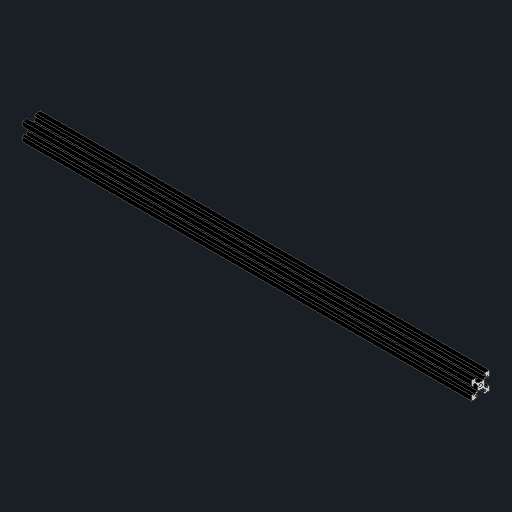
# Autodesk Inventor part: V Extrustion 20x500mm
Saved by Autodesk Inventor 2025.1 (Build 291241000, 241)
## iProperties
Created: 2024-10-17
Part Number: V Extrustion 20x500mm
Material: Generic
Document SubType Name: Modeling
Designer: jerem
Density: 1 g/cm^3
Appearance: Default
Author: jerem
Autodesk Inventor part; units mm, degrees
ref_plane "YZ Plane" through (0, 0, 0) normal (1, 0, 0) x (0, 1, 0)
ref_plane "XZ Plane" through (0, 0, 0) normal (0, 1, 0) x (-1, 0, 0)
ref_plane "XY Plane" through (0, 0, 0) normal (0, 0, 1) x (1, 0, 0)
sketch "Sketch1" plane through (0, 0, 0) normal (1, 0, 0) x (0, 1, 0)
  line L0 (-9.95, -9.95) -> (9.95, -9.95) construction
  line L1 (9.95, 9.95) -> (-9.95, 9.95) construction
  line L2 (-9.95, 9.95) -> (-9.95, -9.95) construction
  line L3 (-9.95, -9.95) -> (9.95, 9.95) construction
  line L4 (9.95, -9.95) -> (-9.95, 9.95) construction
  line L5 (9.95, 4.925) -> (8.15, 3.125)
  line L6 (8.15, 3.125) -> (8.15, 5.4393)
  line L7 (8.15, 5.4393) -> (6.5, 5.4393)
  line L8 (6.5, 5.4393) -> (3.9107, 2.85)
  line L9 (3.9107, 2.85) -> (3.9107, 0)
  line L10 (9.95, -4.925) -> (8.15, -3.125)
  line L11 (8.15, -3.125) -> (8.15, -5.4393)
  line L12 (3.9107, -2.85) -> (3.9107, 0)
  line L13 (0, 0) -> (6.8658, 0) construction
  line L14 (8.15, -5.4393) -> (6.5, -5.4393)
  line L15 (6.5, -5.4393) -> (3.9107, -2.85)
  circle A0 centre (0, 0) radius 2
  line L16 (9.95, -9.95) -> (9.95, -4.925)
  line L17 (9.95, 4.925) -> (9.95, 9.95)
  line L18 (-4.925, 9.95) -> (-9.95, 9.95)
  line L19 (-4.925, 9.95) -> (-3.125, 8.15)
  line L20 (-5.4393, 6.5) -> (-2.85, 3.9107)
  line L21 (-5.4393, 8.15) -> (-5.4393, 6.5)
  line L22 (-3.125, 8.15) -> (-5.4393, 8.15)
  line L23 (-2.85, 3.9107) -> (0, 3.9107)
  line L24 (2.85, 3.9107) -> (0, 3.9107)
  line L25 (5.4393, 6.5) -> (2.85, 3.9107)
  line L26 (5.4393, 8.15) -> (5.4393, 6.5)
  line L27 (3.125, 8.15) -> (5.4393, 8.15)
  line L28 (4.925, 9.95) -> (3.125, 8.15)
  line L29 (9.95, 9.95) -> (4.925, 9.95)
  line L30 (-9.95, -4.925) -> (-9.95, -9.95)
  line L31 (-9.95, -4.925) -> (-8.15, -3.125)
  line L32 (-6.5, -5.4393) -> (-3.9107, -2.85)
  line L33 (-8.15, -5.4393) -> (-6.5, -5.4393)
  line L34 (-8.15, -3.125) -> (-8.15, -5.4393)
  line L35 (-3.9107, -2.85) -> (-3.9107, 0)
  line L36 (-3.9107, 2.85) -> (-3.9107, 0)
  line L37 (-6.5, 5.4393) -> (-3.9107, 2.85)
  line L38 (-8.15, 5.4393) -> (-6.5, 5.4393)
  line L39 (-8.15, 3.125) -> (-8.15, 5.4393)
  line L40 (-9.95, 4.925) -> (-8.15, 3.125)
  line L41 (-9.95, 9.95) -> (-9.95, 4.925)
  line L42 (4.925, -9.95) -> (9.95, -9.95)
  line L43 (4.925, -9.95) -> (3.125, -8.15)
  line L44 (5.4393, -6.5) -> (2.85, -3.9107)
  line L45 (5.4393, -8.15) -> (5.4393, -6.5)
  line L46 (3.125, -8.15) -> (5.4393, -8.15)
  line L47 (2.85, -3.9107) -> (0, -3.9107)
  line L48 (-2.85, -3.9107) -> (0, -3.9107)
  line L49 (-5.4393, -6.5) -> (-2.85, -3.9107)
  line L50 (-5.4393, -8.15) -> (-5.4393, -6.5)
  line L51 (-3.125, -8.15) -> (-5.4393, -8.15)
  line L52 (-4.925, -9.95) -> (-3.125, -8.15)
  line L53 (-9.95, -9.95) -> (-4.925, -9.95)
  dimension "d0" = 19.9
  dimension "d1" = 19.9
  dimension "d3" = 6.25
  dimension "d4" = 5.7
  dimension "d5" = 0.75
  dimension "d7" = 4
  dimension "d8" = 1.8
  dimension "d9" = 45
  dimension "d10" = 1.65
  dimension "d13" = 360
  constraints: 108 end point, 6 parallel, 5 equal length, 3 horizontal, 3 perpendicular, 3 vertical, 2 midpoint, 1 centre point, 1 coincident, 1 point on line, 101 other
  measures "d0" distance of L1.end L1.start
  measures "d1" distance of L1.start L0.end
  measures "d3" distance of L10.end L5.end
  measures "d4" distance of L12.start L8.end
  measures "d5" distance between parallel lines of L3 L8
  measures "d7" diameter of A0
  measures "d8" distance between parallel lines of L6 L17
  measures "d9" angle of L6 L5
  measures "d10" distance from line of L7.end L6
extrude "Extrusion1" add sketch "Sketch1" along normal blind 500
body "Solid1"
